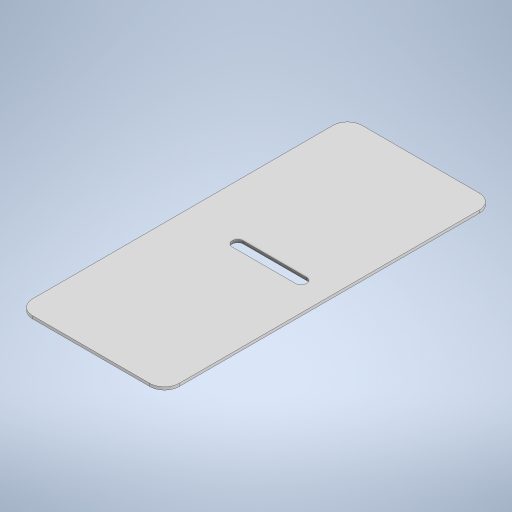
# Autodesk Inventor part: Module PCB Edge Clip
Saved by Autodesk Inventor 2023 (Build 270158000, 158)
## iProperties
Created: 2022-11-30
Part Number: Module PCB Edge Clip
Material: Generic
Document SubType Name: Modeling
Designer: Caleb
Density: 1 g/cm^3
Appearance: Default
Author: Caleb
Autodesk Inventor part; units mm, degrees
ref_plane "YZ Plane" through (0, 0, 0) normal (1, 0, 0) x (0, 1, 0)
ref_plane "XZ Plane" through (0, 0, 0) normal (0, 1, 0) x (-1, 0, 0)
ref_plane "XY Plane" through (0, 0, 0) normal (0, 0, 1) x (1, 0, 0)
sketch "Sketch1" plane through (0, 0, 0) normal (0, 1, 0) x (-1, 0, 0)
  line L0 (-8, -22.5) -> (8, -22.5)
  line L1 (10, -20.5) -> (10, 20.5)
  line L2 (8, 22.5) -> (-8, 22.5)
  line L3 (-10, 20.5) -> (-10, -20.5)
  line L4 (-10, -22.5) -> (10, 22.5) construction
  line L5 (10, -22.5) -> (-10, 22.5) construction
  arc A0 (10, 20.5) -> (8, 22.5) centre (8, 20.5) ccw
  arc A1 (-8, 22.5) -> (-10, 20.5) centre (-8, 20.5) ccw
  arc A2 (-10, -20.5) -> (-8, -22.5) centre (-8, -20.5) ccw
  arc A3 (8, -22.5) -> (10, -20.5) centre (8, -20.5) ccw
  point P0 (0, 0)
  dimension "d0" = 45
  dimension "d1" = 20
  dimension "d2" = 2
  constraints: 12 end point, 8 point on circle, 8 point on line, 8 tangent, 4 centre point, 3 equal radius, 2 midpoint, 2 parallel, 1 horizontal, 1 perpendicular
  measures "d0" distance of L5.start L4.end
  measures "d1" distance of L4.end L5.end
  measures "d2" radius of A0
extrude "Extrusion1" add sketch "Sketch1" along normal blind 0.381
sketch "Sketch2" plane through (0, 0.381, 0) normal (0, 1, 0) x (1, 0, 0)
  line L0 (-2.4882, 0) -> (6.1489, 0) construction
  line L1 (-2.4882, -0.7436) -> (6.1489, -0.7436)
  line L2 (6.1489, 0.7436) -> (-2.4882, 0.7436)
  arc A0 (-2.4882, 0.7436) -> (-2.4882, -0.7436) centre (-2.4882, 0) ccw
  arc A1 (6.1489, -0.7436) -> (6.1489, 0.7436) centre (6.1489, 0) ccw
  point P0 (0, 0)
  point P1 (1.8304, 0)
  constraints: 8 end point, 4 point on circle, 4 tangent, 2 centre point, 1 horizontal, 1 midpoint, 1 parallel
extrude "Extrusion2" cut sketch "Sketch2" against normal through all
body "Solid1"
